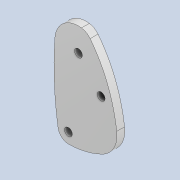
# Autodesk Inventor part: アンノーン後
Saved by Autodesk Inventor 2020.4 (Build 244396000, 396)
## iProperties
Created: 2021-02-23
Part Number: アンノーン後
Material: アルミニウム 2014-T4
Document SubType Name: Modeling
Designer: AA19065
Density: 2.8 g/cm^3
Appearance: サテン
Mass: 6.96629 g
Surface Area: 21.5315 cm^2
Volume: 2.48796 cm^3
Author: AA19065
Autodesk Inventor part; units mm, degrees
ref_plane "YZ Plane" through (0, 0, 0) normal (1, 0, 0) x (0, 1, 0)
ref_plane "XZ Plane" through (0, 0, 0) normal (0, 1, 0) x (-1, 0, 0)
ref_plane "XY Plane" through (0, 0, 0) normal (0, 0, 1) x (1, 0, 0)
sketch "スケッチ1" plane through (0, 0, 0) normal (0, 0, 1) x (1, 0, 0)
  line L0 (108, 72.8318) -> (108, -27.6373) construction
  circle A0 centre (90, 27) radius 3
  circle A1 centre (104.0735, 2) radius 6.025
  circle A2 centre (90, 27) radius 1.5
  circle A3 centre (104.0735, 2) radius 1.5
  circle A4 centre (82.0403, 11.2819) radius 1.5
  circle A5 centre (82.5, -8) radius 3
  circle A6 centre (82.5, -8) radius 1.5
  arc A7 (66.6452, -5.64) -> (72.9159, -4.36) centre (69.7806, -5) ccw
  arc A8 (72.7246, 23.8286) -> (66.6452, -5.64) centre (104.0735, 2) ccw
  arc A9 (77.9767, 20.1714) -> (72.9159, -4.36) centre (104.0735, 2) ccw
  arc A10 (77.9767, 20.1714) -> (72.7246, 23.8286) centre (75.3506, 22) ccw
  circle A11 centre (137.3222, 20) radius 1.25
  circle A12 centre (133.5, -8) radius 3
  circle A13 centre (133.5, -8) radius 1.5
  circle A14 centre (146, 10) radius 1.5
  arc A15 (-6.0896, 13.373) -> (73.9904, 1.933) centre (42.2887, 66.0206) ccw construction
  line L1 (108, 72.8318) -> (108, -27.6373) construction
  arc A16 (142.0096, 1.933) -> (222.0896, 13.373) centre (173.7113, 66.0206) ccw construction
  arc A17 (142.297, -19.0729) -> (142.6609, 27.2536) centre (125.7093, 4.222) ccw
  arc A18 (136.8078, 35.1273) -> (180.0662, 10.7187) centre (180.8617, 62.6652) ccw
  circle A19 centre (137.3222, 20) radius 9.0064
  arc A20 (128.3227, 20.3537) -> (130.5559, -8.5765) centre (253.2262, 15.4443) ccw
  arc A21 (133.4146, -10.9988) -> (152.9487, -4.4855) centre (134.2687, 18.9891) ccw
  arc A22 (35.9338, 10.7187) -> (79.1922, 35.1273) centre (35.1383, 62.6652) ccw
  arc A23 (73.3391, 27.2536) -> (73.703, -19.0729) centre (90.2907, 4.222) ccw
  arc A24 (90.8877, 29.8657) -> (71.1185, 25.1885) centre (84.9697, 10.7613) ccw
  arc A25 (109.5592, 4.4914) -> (92.0759, 29.1658) centre (36.7191, -28.5891) ccw
  arc A26 (80.5672, -10.2944) -> (70.6533, -16.5669) centre (76.6032, -15) ccw
  circle A27 centre (76.6032, -15) radius 5 construction
  circle A28 centre (94, -11) radius 1.5
  circle A29 centre (94, -11) radius 3
  arc A30 (103.1113, -3.9477) -> (84.6572, -10.0848) centre (99.758, -24.6782) ccw
  line L2 (108, 72.8318) -> (108, -27.6373) construction
  circle A31 centre (90, 27) radius 3
  circle A32 centre (104.0735, 2) radius 6.025
  circle A33 centre (90, 27) radius 1.5
  circle A34 centre (104.0735, 2) radius 1.5
  circle A35 centre (82.0403, 11.2819) radius 1.5
  circle A36 centre (82.5, -8) radius 3
  circle A37 centre (82.5, -8) radius 1.5
  arc A38 (66.6452, -5.64) -> (72.9159, -4.36) centre (69.7806, -5) ccw
  arc A39 (72.7246, 23.8286) -> (66.6452, -5.64) centre (104.0735, 2) ccw
  arc A40 (77.9767, 20.1714) -> (72.9159, -4.36) centre (104.0735, 2) ccw
  arc A41 (77.9767, 20.1714) -> (72.7246, 23.8286) centre (75.3506, 22) ccw
  circle A42 centre (137.3222, 20) radius 1.25
  circle A43 centre (133.5, -8) radius 4
  circle A44 centre (133.5, -8) radius 1.5
  circle A45 centre (146, 10) radius 1.5
  arc A46 (-6.0896, 13.373) -> (73.9904, 1.933) centre (42.2887, 66.0206) ccw construction
  line L3 (108, 72.8318) -> (108, -27.6373) construction
  arc A47 (142.0096, 1.933) -> (222.0896, 13.373) centre (173.7113, 66.0206) ccw construction
  arc A48 (142.297, -19.0729) -> (142.6609, 27.2536) centre (125.7093, 4.222) ccw
  arc A49 (136.8078, 35.1273) -> (180.0662, 10.7187) centre (180.8617, 62.6652) ccw
  circle A50 centre (137.3222, 20) radius 9.0064
  arc A51 (128.342, 20.688) -> (129.5504, -8.6327) centre (252.9768, 11.1391) ccw
  arc A52 (133.5638, -11.9995) -> (152.9487, -4.4855) centre (133.0855, 17.9967) ccw
  arc A53 (35.9338, 10.7187) -> (79.1922, 35.1273) centre (35.1383, 62.6652) ccw
  arc A54 (73.3391, 27.2536) -> (73.703, -19.0729) centre (90.2907, 4.222) ccw
  arc A55 (90.8877, 29.8657) -> (71.1185, 25.1885) centre (84.9697, 10.7613) ccw
  arc A56 (109.5592, 4.4914) -> (92.0759, 29.1658) centre (36.7191, -28.5891) ccw
  arc A57 (80.5672, -10.2944) -> (70.6533, -16.5669) centre (76.6032, -15) ccw
  circle A58 centre (76.6032, -15) radius 5 construction
  circle A59 centre (94, -11) radius 1.5
  circle A60 centre (94, -11) radius 3
  arc A61 (103.1113, -3.9477) -> (84.6572, -10.0848) centre (99.758, -24.6782) ccw
  circle A62 centre (137.3222, 20) radius 1.5
  point P0 (0, 0)
  point P1 (0, 0)
  point P2 (0, 0)
  point P3 (153.4907, -2.5604)
  point P4 (70.4206, -8.1353)
  point P5 (68.8141, 23.1049)
  point P6 (143.7549, 26.3036)
  point P7 (147.1859, 23.1049)
  point P8 (0, 0)
  point P9 (153.4907, -2.5604)
  point P10 (152.9487, -4.4855)
  dimension "d0" = 2
  dimension "d1" = 30
  dimension "d2" = 125
  dimension "d3" = 80
  dimension "d4" = 20
  dimension "d5" = 6
  dimension "d6" = 21
  dimension "d14" = 2
  dimension "d15" = 30
  dimension "d16" = 125
  dimension "d17" = 80
  dimension "d18" = 20
  dimension "d19" = 6
  dimension "d20" = 21
  dimension "d25" = 3
  constraints: 93 point on circle, 61 centre point, 20 tangent, 8 end point, 6 symmetric about line, 3 coincident, 1 vertical, 40 other
  measures "d0" distance of point (153.491, -2.56) A21.end
  measures "d1" radius of A21
  measures "d2" radius of A20
  measures "d3" radius of A25
  measures "d4" radius of A24
  measures "d5" diameter of A29
  measures "d6" radius of A30
  measures "d14" distance of point (153.491, -2.56) A52.end
  measures "d15" radius of A52
  measures "d16" radius of A51
  measures "d17" radius of A56
  measures "d18" radius of A55
  measures "d19" diameter of A60
  measures "d20" radius of A61
  measures "d25" diameter of A62
extrude "押し出し1" add sketch "スケッチ1" along normal blind 3 contours A12 | A12 A20 A43 A21 | A12 A21 A43 A20 | A43 A51 A19 A20 | A20 A19 A18 A17 A21 A43 | A21 A52 A43 | A19
fillet "フィレット1" radius 3 1 edges at (152.9487, -4.4855, 1.5)
fillet "フィレット2" radius 5 1 edges at (147.1859, 23.1049, 1.5)
sketch "スケッチ3" plane through (0, 0, 0) normal (0, 0, -1) x (-1, 0, 0)
  arc A0 (-146.9178, 23.3347) -> (-147.4526, 22.7972) centre (-143.6509, 19.5495) ccw projected
  arc A1 (-147.4526, 22.7972) -> (-153.2165, -3.5986) centre (-125.7093, 4.222) ccw projected
  arc A2 (-152.247, -5.0865) -> (-133.5638, -11.9995) centre (-133.0855, 17.9967) ccw projected
  arc A3 (-133.5638, -11.9995) -> (-129.5504, -8.6327) centre (-133.5, -8) ccw projected
  arc A4 (-129.5504, -8.6327) -> (-128.342, 20.688) centre (-252.9768, 11.1391) ccw projected
  arc A5 (-128.342, 20.688) -> (-143.7549, 26.3036) centre (-137.3222, 20) ccw projected
  arc A6 (-146.9178, 23.3347) -> (-143.7549, 26.3036) centre (-180.8617, 62.6652) ccw projected
  circle A7 centre (-133.5, -8) radius 1.5 projected
  circle A8 centre (-146, 10) radius 1.5 projected
  circle A9 centre (-137.3222, 20) radius 3.1
  circle A10 centre (-146, 10) radius 3.1
  circle A11 centre (-133.5, -8) radius 3.1
  arc A12 (-153.2165, -3.5986) -> (-152.247, -5.0865) centre (-150.3308, -2.7782) ccw projected
  circle A13 centre (-137.3222, 20) radius 1.5 projected
  point P0 (0, 0)
  dimension "d21" = 6.2
  dimension "d22" = 6.2
  dimension "d23" = 6.2
  constraints: 3 centre point, 2 coincident, 1 concentric
  measures "d21" diameter of A9
  measures "d22" diameter of A10
  measures "d23" diameter of A11
extrude "押し出し2" cut sketch "スケッチ3" against normal blind 1 contours A9 | A10 | A11
sketch "スケッチ4" plane through (0, 0, 3) normal (0, 0, 1) x (1, 0, 0)
  arc A0 (147.4526, 22.7972) -> (146.9178, 23.3347) centre (143.6509, 19.5495) ccw projected
  arc A1 (143.7549, 26.3036) -> (146.9178, 23.3347) centre (180.8617, 62.6652) ccw projected
  arc A2 (143.7549, 26.3036) -> (128.342, 20.688) centre (137.3222, 20) ccw projected
  arc A3 (128.342, 20.688) -> (129.5504, -8.6327) centre (252.9768, 11.1391) ccw projected
  arc A4 (129.5504, -8.6327) -> (133.5638, -11.9995) centre (133.5, -8) ccw projected
  arc A5 (133.5638, -11.9995) -> (152.247, -5.0865) centre (133.0855, 17.9967) ccw projected
  arc A6 (152.247, -5.0865) -> (153.2165, -3.5986) centre (150.3308, -2.7782) ccw projected
  arc A7 (153.2165, -3.5986) -> (147.4526, 22.7972) centre (125.7093, 4.222) ccw projected
  circle A8 centre (146, 10) radius 1.5 projected
  circle A9 centre (137.3222, 20) radius 1.5 projected
  circle A10 centre (133.5, -8) radius 1.5 projected
  arc A11 (153.2165, -3.5986) -> (147.4526, 22.7972) centre (125.7093, 4.222) ccw projected
  arc A12 (143.7549, 26.3036) -> (128.342, 20.688) centre (137.3222, 20) ccw projected
  spline S0 degree 2 poles (140.7582, 28.3253) (151.7544, 15.1223) (152.5321, -5.695) knots 0 0 0 1 1 1
  circle A13 centre (146, 10) radius 3.1 projected
  point P0 (0, 0)
  point P1 (148.8945, 14.077)
  point P2 (140.7582, 28.3253)
  point P3 (153.3615, -3.0694)
  point P4 (152.4964, -4.8544)
  dimension "d36" = 5
  dimension "d37" = 13
  dimension "d38" = 17
  dimension "d39" = 36
  constraints: 2 point on circle, 3 other
  measures "d36" distance of A8.centre point (148.894, 14.077)
  measures "d37" distance of A9.centre point (148.894, 14.077)
  measures "d38" distance of A8.centre point (152.532, -5.695)
  measures "d39" distance of point (152.532, -5.695) point (140.758, 28.325)
extrude "押し出し3" cut sketch "スケッチ4" against normal blind 10 contours A7 A6 S0 A2 A1 A0
fillet "フィレット3" radius 10 1 edges at (152.4964, -4.8544, 1.5)
fillet "フィレット4" radius 5 1 edges at (140.7582, 28.3253, 1.5)
